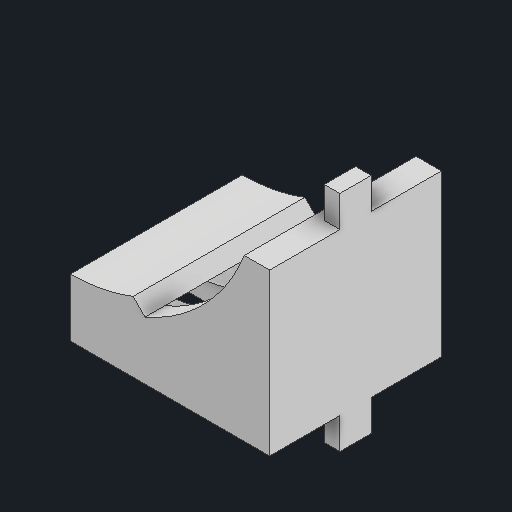
# Autodesk Inventor part: Piece-Catch
Saved by Autodesk Inventor 2025 (Build 290162010, 162A)
## iProperties
Created: 2025-12-06
Part Number: Piece-Catch
Material: Generic
Document SubType Name: Modeling
Designer: FizzyApple12
Density: 1 g/cm^3
Appearance: Default
Author: FizzyApple12
Autodesk Inventor part; units mm, degrees
ref_plane "YZ Plane" through (0, 0, 0) normal (1, 0, 0) x (0, 1, 0)
ref_plane "XZ Plane" through (0, 0, 0) normal (0, 1, 0) x (-1, 0, 0)
ref_plane "XY Plane" through (0, 0, 0) normal (0, 0, 1) x (1, 0, 0)
sketch "Sketch1" plane through (0, 0, 0) normal (0, 0, 1) x (1, 0, 0)
  line L0 (0, 0) -> (-53, 0)
  line L1 (-53, 0) -> (-53, 33.25) construction
  line L2 (-53, 33.25) -> (0, 33.25)
  line L3 (0, 33.25) -> (0, 0)
  line L4 (-51, 33.25) -> (-51, 0)
  line L5 (0, 0) -> (-51, 0)
  line L6 (-51, 0) -> (-51, -4)
  line L7 (-51, -4) -> (0, -4)
  line L8 (0, -4) -> (0, 0)
  circle A0 centre (-51, 54.6729) radius 54.6729
  line L9 (-26.7487, 5.6729) -> (-2, 30.4216)
  line L10 (-2, 30.4216) -> (-4.8284, 33.25)
  line L11 (-4.8284, 33.25) -> (-29.5772, 8.5013)
  line L12 (-29.5772, 8.5013) -> (-26.7487, 5.6729) construction
  circle A1 centre (-51, 54.6729) radius 47.7965
  line L13 (-29.5772, 8.5013) -> (-31.924, 10.8481)
  circle A2 centre (-51, 54.6729) radius 43.7965
  line L14 (-31.924, 10.8481) -> (-34.9853, 13.9094)
  line L15 (-51, 33.25) -> (0, 33.25)
  line L16 (0, 33.25) -> (0, 37.25)
  line L17 (0, 37.25) -> (-51, 37.25)
  line L18 (-51, 37.25) -> (-51, 33.25)
  line L19 (-4.8284, 33.25) -> (-8.8284, 37.25)
  point P0 (-51, 10.8764)
  point P1 (-51, 6.8764)
  point P2 (-8.2734, 33.25)
  point P3 (-6.4922, 37.25)
  point P4 (-7.1753, 35.5969)
  point P5 (-0.699, 33.25)
  point P6 (0, 34.972)
  dimension "d22" = 95.5929
  dimension "d23" = 87.5929
  dimension "d0" = 53
  dimension "d5" = 51
  dimension "d13" = 4
  dimension "d18" = 35
  dimension "d19" = 4
  dimension "d20" = 2
  dimension "d21" = 45
  dimension "d24" = 4
  constraints: 40 end point, 8 parallel, 5 perpendicular, 4 point on line, 3 collinear, 3 horizontal, 3 point on circle, 2 coincident, 1 centre point, 1 tangent, 7 other
  measures "d0" distance of L1.end L2.end
  measures "d5" distance between parallel lines of L3 L4
  measures "d13" distance between parallel lines of L7 L0
  measures "d18" distance of L9.start L9.end
  measures "d19" distance of L10.end L9.end
  measures "d20" distance from line of L9.end L3
  measures "d21" angle of L3 L9
  measures "d24" distance of L2.end L16.end
extrude "Extrusion1" add sketch "Sketch1" along normal blind 44 contours L8 L7 L6 L0 | L0 A0 L2 L3 | L2 A0 L16 | L4 A2 L14 A1 | A0 L10 L2 | L2 L19 A1 L17 L16 A0
extrude "Extrusion2" add sketch "Sketch1" along normal blind 5 contours L8 L7 L6 L0 | L0 A0 L2 L3 | L4 A1 L13 L11 L10 L9 A0 | L4 A2 L14 A1 | L9 A0 | A0 L10 L2 | A1 L11 L13 | L11 A1 L2 | L2 A1 L19
extrude "Extrusion3" add sketch "Sketch1" against normal blind 5 from surface at 44 contours L0 A0 L2 L3 | L4 A1 L13 L11 L10 L9 A0 | L4 A2 L14 A1 | L9 A0 | A0 L10 L2 | L2 L19 A1 L17 L16 A0 | A1 L11 L13 | L11 A1 L2 | L2 A1 L19
sketch "Sketch3" plane through (0, -4, 0) normal (1, 0, 0) x (0, 0, -1)
  line L0 (0, 0) -> (0, 41.25) construction
  line L1 (0, 41.25) -> (-44, 41.25) construction
  line L2 (-44, 0) -> (-44, 41.25) construction
  line L3 (0, 0) -> (-44, 0) construction
  line L4 (-26, 0) -> (-18, 0)
  line L5 (-18, 0) -> (-18, -8)
  line L6 (-18, -8) -> (-26, -8)
  line L7 (-26, -8) -> (-26, 0)
  line L8 (-26, 49.25) -> (-18, 49.25)
  line L9 (-18, 49.25) -> (-18, 41.25)
  line L10 (-18, 41.25) -> (-26, 41.25)
  line L11 (-26, 41.25) -> (-26, 49.25)
  line L12 (-26, 0) -> (-18, -8) construction
  line L13 (-26, 49.25) -> (-18, 41.25) construction
  point P0 (0, 4)
  point P1 (-22, 0)
  point P2 (-22, 41.25)
  point P3 (-22, -4)
  point P4 (-22, 45.25)
  dimension "d33" = 8
  dimension "d34" = 8
  dimension "d35" = 8
  dimension "d36" = 8
  constraints: 20 end point, 6 midpoint, 4 parallel, 2 horizontal, 2 perpendicular
  measures "d33" distance of L5.end L6.end
  measures "d34" distance of L4.end L5.end
  measures "d35" distance of L9.end L10.end
  measures "d36" distance of L8.end L9.end
extrude "Extrusion5" add sketch "Sketch3" against normal blind 4
sketch "Sketch2" plane through (-51, -4, 0) normal (0, -1, 0) x (1, 0, 0)
  line L0 (30, 26) -> (0, 26)
  line L1 (0, 26) -> (0, 18)
  line L2 (0, 18) -> (30, 18)
  line L3 (30, 18) -> (30, 26)
  line L4 (0, 0) -> (0, 44) construction
  point P0 (51, 0)
  point P1 (0, 22)
  dimension "d29" = 30
  dimension "d30" = 8
  constraints: 8 end point, 2 midpoint, 2 parallel, 1 horizontal, 1 perpendicular
  measures "d29" distance of L2.end L1.end
  measures "d30" distance of L1.end L0.end
extrude "Extrusion4" cut sketch "Sketch2" against normal up to surface
fillet "Fillet2" [suppressed]
chamfer "Chamfer2" [suppressed]
body "Solid1"
